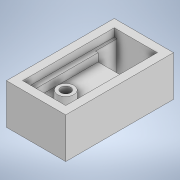
# Autodesk Inventor part: Holder
Saved by Autodesk Inventor 2020 (Build 240168000, 168)
## iProperties
Created: 2019-07-08
Part Number: Holder
Material: Generic
Document SubType Name: Modeling
Designer: simon
Density: 1 g/cm^3
Appearance: Default
Author: simon
Autodesk Inventor part; units mm, degrees
ref_plane "YZ Plane" through (0, 0, 0) normal (1, 0, 0) x (0, 1, 0)
ref_plane "XZ Plane" through (0, 0, 0) normal (0, 1, 0) x (-1, 0, 0)
ref_plane "XY Plane" through (0, 0, 0) normal (0, 0, 1) x (1, 0, 0)
sketch "Sketch1" plane through (0, 0, 0) normal (0, 1, 0) x (-1, 0, 0)
  line L0 (11, 20) -> (-11, 20)
  line L1 (-11, 20) -> (-11, -20)
  line L2 (-11, -20) -> (11, -20)
  line L3 (11, -20) -> (11, 20)
  line L4 (11, 20) -> (-11, -20) construction
  line L5 (-11, 20) -> (11, -20) construction
  dimension "d0" = 22
  dimension "d1" = 40
  constraints: 12 end point, 2 parallel, 1 horizontal, 1 perpendicular
  measures "d0" distance of L2.end L1.end
  measures "d1" distance of L1.end L0.end
extrude "Extrusion1" add sketch "Sketch1" along normal blind 15
sketch "Sketch2" plane through (0, 15, 0) normal (0, 1, 0) x (1, 0, 0)
  line L0 (-8, -17) -> (8, -17)
  line L1 (8, -17) -> (8, 17)
  line L2 (8, 17) -> (-8, 17)
  line L3 (-8, 17) -> (-8, -17)
  line L4 (-8, -17) -> (8, 17) construction
  line L5 (8, -17) -> (-8, 17) construction
  point P0 (0, 0)
  dimension "d6" = 16
  dimension "d7" = 34
  constraints: 12 end point, 2 midpoint, 2 parallel, 1 horizontal, 1 perpendicular
  measures "d6" distance of L2.end L1.end
  measures "d7" distance of L1.end L0.end
extrude "Extrusion2" cut sketch "Sketch2" against normal blind 3
sketch "Sketch3" plane through (0, 12, 0) normal (0, 1, 0) x (1, 0, 0)
  line L0 (6, -17) -> (-6, -17)
  line L1 (-6, -17) -> (-6, 17)
  line L2 (-6, 17) -> (6, 17)
  line L3 (6, 17) -> (6, -17)
  line L4 (6, -17) -> (-6, 17) construction
  line L5 (-6, -17) -> (6, 17) construction
  point P0 (0, 0)
  dimension "d10" = 12
  dimension "d11" = 34
  constraints: 12 end point, 2 midpoint, 2 parallel, 1 horizontal, 1 perpendicular
  measures "d10" distance of L1.end L2.end
  measures "d11" distance of L0.end L1.end
extrude "Extrusion3" cut sketch "Sketch3" against normal blind 3
sketch "Sketch4" plane through (0, 15, 0) normal (0, 1, 0) x (1, 0, 0)
  line L0 (-7, 9) -> (7, 9)
  line L1 (7, 9) -> (7, 17)
  line L2 (7, 17) -> (-7, 17)
  line L3 (-7, 17) -> (-7, 9)
  line L4 (-7, 9) -> (7, 17) construction
  line L5 (7, 9) -> (-7, 17) construction
  point P0 (0, 0)
  point P1 (0, 13)
  dimension "d14" = 14
  dimension "d15" = 8
  constraints: 12 end point, 2 midpoint, 2 parallel, 1 horizontal, 1 perpendicular
  measures "d14" distance of L2.end L1.end
  measures "d15" distance of L1.end L0.end
extrude "Extrusion4" cut sketch "Sketch4" against normal through all
sketch "Sketch5" plane through (0, 9, 0) normal (0, 1, 0) x (1, 0, 0)
  circle A0 centre (0, -9) radius 3
  point P0 (0, 0)
  dimension "d18" = 6
  constraints: 1 centre point
  measures "d18" diameter of A0
extrude "Extrusion5" add sketch "Sketch5" along normal up to surface (3 mm away)
sketch "Sketch6" plane through (0, 12, 9) normal (0, 1, 0) x (1, 0, 0)
  point P0 (0, 9)
  point P1 (0, 0)
  point P2 (0, 0)
  constraints: 1 coincident
hole "Hole1" at (0, 12, 9) direction (0, -1, 0) diameter 3.6 end through all clearance for "Socket Head Cap Screw DIN EN ISO 4762" size "M3" standard "DIN"
sketch "Sketch7" plane through (0, 0, 0) normal (0, -1, 0) x (1, 0, 0)
  circle A0 centre (0, 9) radius 1.8 projected
  line L0 (1.7032, 11.95) -> (3.4064, 9)
  line L1 (3.4064, 9) -> (1.7032, 6.05)
  line L2 (1.7032, 6.05) -> (-1.7032, 6.05)
  line L3 (-1.7032, 6.05) -> (-3.4064, 9)
  line L4 (-3.4064, 9) -> (-1.7032, 11.95)
  line L5 (-1.7032, 11.95) -> (1.7032, 11.95)
  point P0 (0, 0)
  point P1 (0, 11.95)
  constraints: 12 end point, 2 coincident, 1 midpoint, 13 other
extrude "Extrusion6" cut sketch "Sketch7" against normal blind 5
body "Solid1"
